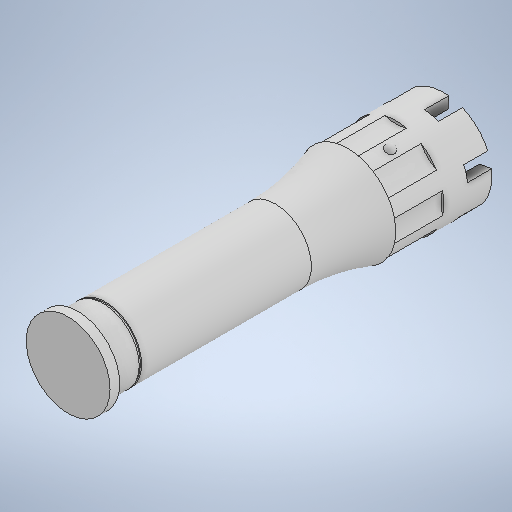
# Autodesk Inventor part: Capsule idea
Saved by Autodesk Inventor 2026.2 (Build 302298000, 298)
## iProperties
Created: 2026-01-17
Part Number: Capsule idea
Material: Generic
Document SubType Name: Modeling
Designer: daryu
Density: 1 g/cm^3
Appearance: Default
Author: daryu
Autodesk Inventor part; units mm, degrees
ref_plane "YZ Plane" through (0, 0, 0) normal (1, 0, 0) x (0, 1, 0)
ref_plane "XZ Plane" through (0, 0, 0) normal (0, 1, 0) x (-1, 0, 0)
ref_plane "XY Plane" through (0, 0, 0) normal (0, 0, 1) x (1, 0, 0)
sketch "Sketch2" plane through (0, 0, 0) normal (1, 0, 0) x (0, 1, 0)
  line L0 (0, 0) -> (15, 0)
  line L1 (15, 0) -> (15, -50)
  line L2 (15, -50) -> (0, -50)
  line L3 (0, -50) -> (0, 0)
  line L4 (7.5, 0) -> (7.5, -50)
  dimension "d0" = 50
  dimension "d1" = 15
  constraints: 10 end point, 2 midpoint, 2 parallel, 2 perpendicular, 1 horizontal
  measures "d0" distance of L0.end L1.end
  measures "d1" distance of L0.start L0.end
revolve "Revolution1" add sketch "Sketch2" angle 360 about axis through (0, 7.5, 0) along (0, 0, -1) contours L0 L1 L2 L4
sketch "Sketch3" plane through (0, 0, 0) normal (1, 0, 0) x (0, 1, 0)
  line L0 (0, -50) -> (15, -50) projected
  line L1 (0, -50) -> (0, -43)
  line L2 (0, 0) -> (0, -50) projected
  arc A0 (-2.5, -58) -> (0, -43) centre (-46.25, -43) ccw
  line L3 (-2.5, -58) -> (0, -58)
  line L4 (0, -58) -> (0, -50)
  line L5 (0, 0) -> (15, 0) projected
  line L6 (7.5, 0) -> (7.5, -50)
  dimension "d5" = 15
  dimension "d6" = 2.5
  dimension "d7" = 8
  constraints: 8 end point, 2 midpoint, 2 point on circle, 1 centre point, 1 horizontal, 1 horizontal alignment, 1 perpendicular, 1 point on line
  measures "d5" vertical distance of L1.end L3.start
  measures "d6" distance of L3.start L3.end
  measures "d7" distance of L0.start L3.end
revolve "Revolution2" add sketch "Sketch3" angle 360 about axis through (0, 7.5, 0) along (0, 0, -1) contours L4 L3 A0 L1
sketch "Sketch4" plane through (0, 7.5, -58) normal (0, 0, -1) x (-1, 0, 0)
  circle A0 centre (0, 0) radius 10 projected
  point P0 (0, -7.5)
extrude "Extrusion1" add sketch "Sketch4" along normal blind 10
sketch "Sketch5" plane through (0, 7.5, -68) normal (0, 0, -1) x (-1, 0, 0)
  circle A0 centre (0, 0) radius 10 projected
  line L0 (0, 0) -> (0, -3.294)
  line L1 (0, 0) -> (7.0711, 7.0711)
  line L2 (0, 0) -> (0, 10)
  arc A1 (5.2892, 8.4867) -> (8.4867, 5.2892) centre (11.8815, 11.8815) ccw
  arc A2 (-2.261, 9.741) -> (2.261, 9.741) centre (0, 16.803) ccw
  arc A3 (-8.4867, 5.2892) -> (-5.2892, 8.4867) centre (-11.8815, 11.8815) ccw
  arc A4 (-9.741, -2.261) -> (-9.741, 2.261) centre (-16.803, 0) ccw
  arc A5 (-5.2892, -8.4867) -> (-8.4867, -5.2892) centre (-11.8815, -11.8815) ccw
  arc A6 (2.261, -9.741) -> (-2.261, -9.741) centre (0, -16.803) ccw
  arc A7 (8.4867, -5.2892) -> (5.2892, -8.4867) centre (11.8815, -11.8815) ccw
  arc A8 (9.741, 2.261) -> (9.741, -2.261) centre (16.803, 0) ccw
  point P0 (0, -7.5)
  point P1 (6.6383, 6.6383)
  point P2 (0, 9.3879)
  point P3 (-6.6383, 6.6383)
  point P4 (-9.3879, 0)
  point P5 (-6.6383, -6.6383)
  point P6 (0, -9.3879)
  point P7 (6.6383, -6.6383)
  point P8 (9.3879, 0)
  point P9 (5.2892, -8.4867)
  point P10 (-2.261, -9.741)
  point P11 (-8.4867, -5.2892)
  point P12 (-9.741, 2.261)
  point P13 (9.741, 2.261)
  point P14 (9.741, -2.261)
  point P15 (2.261, 9.741)
  point P16 (-2.261, 9.741)
  point P17 (-8.4867, 5.2892)
  point P18 (-5.2892, 8.4867)
  dimension "d19" = 3.294
  dimension "d30" = 45
  dimension "d31" = 11.8815
  dimension "d32" = 7.4151
  dimension "d35" = 360
  constraints: 20 point on circle, 8 centre point, 6 end point, 2 vertical, 1 equal length, 1 point on line, 41 other
  measures "d19" distance of L0.start L0.end
  measures "d30" angle of L2 L1
  measures "d31" horizontal distance of L0.start A1.centre
  measures "d32" radius of A1
ref_plane "Work Plane1" through (0, 7.5, 0) normal (0, 0, 1) x (1, 0, 0)
sketch "Sketch6" plane through (0, 7.5, 0) normal (0, 0, 1) x (1, 0, 0)
  circle A0 centre (0, 0) radius 7.5 projected
  circle A1 centre (0, 0) radius 8.7
  point P0 (0, -7.5)
  dimension "d23" = 1.2
  constraints: 1 centre point, 1 vertical alignment
extrude "Extrusion3" add sketch "Sketch6" against normal blind 2
extrude "Extrusion4" cut sketch "Sketch5" against normal blind 10 contours A0 A8 | A1 L1 A0 | A0 A7 | L1 A1 A0 | A0 A6 | A2 L2 A0 | A2 A0 L2 | A0 A5 | A3 A0 | A0 A4
sketch "Sketch7" plane through (0, 7.5, -68) normal (0, 0, -1) x (-1, 0, 0)
  arc A0 (9.741, -2.261) -> (9.741, 2.261) centre (0, 0) ccw projected
  arc A1 (8.4867, -5.2892) -> (9.741, -2.261) centre (0, 0) ccw projected
  arc A2 (5.2892, -8.4867) -> (8.4867, -5.2892) centre (0, 0) ccw projected
  arc A3 (2.261, -9.741) -> (5.2892, -8.4867) centre (0, 0) ccw projected
  arc A4 (-2.261, -9.741) -> (2.261, -9.741) centre (0, 0) ccw projected
  arc A5 (-5.2892, -8.4867) -> (-2.261, -9.741) centre (0, 0) ccw projected
  arc A6 (-8.4867, -5.2892) -> (-5.2892, -8.4867) centre (0, 0) ccw projected
  arc A7 (-9.741, -2.261) -> (-8.4867, -5.2892) centre (0, 0) ccw projected
  arc A8 (-9.741, 2.261) -> (-9.741, -2.261) centre (0, 0) ccw projected
  arc A9 (-8.4867, 5.2892) -> (-9.741, 2.261) centre (0, 0) ccw projected
  arc A10 (-5.2892, 8.4867) -> (-8.4867, 5.2892) centre (0, 0) ccw projected
  arc A11 (-2.261, 9.741) -> (-5.2892, 8.4867) centre (0, 0) ccw projected
  arc A12 (2.261, 9.741) -> (-2.261, 9.741) centre (0, 0) ccw projected
  arc A13 (5.2892, 8.4867) -> (2.261, 9.741) centre (0, 0) ccw projected
  arc A14 (8.4867, 5.2892) -> (5.2892, 8.4867) centre (0, 0) ccw projected
  arc A15 (9.741, 2.261) -> (8.4867, 5.2892) centre (0, 0) ccw projected
  circle A16 centre (0, 0) radius 7.5 projected
  point P0 (0, -7.5)
extrude "Extrusion5" add sketch "Sketch7" along normal blind 10
sketch "Sketch8" plane through (0, 7.5, -78) normal (0, 0, -1) x (-1, 0, 0)
  circle A0 centre (0, 0) radius 7.5 projected
  circle A1 centre (0, 0) radius 10 projected
  line L0 (-4.5, -6) -> (-6.0595, -7.955)
  line L1 (-6, -4.5) -> (-8.1073, -5.8542)
  point P0 (0, -7.5)
  dimension "d41" = 2.5008
  dimension "d42" = 2.5049
  dimension "d43" = 6
  dimension "d44" = 6
  constraints: 4 end point, 4 point on circle
  measures "d41" distance of L0.start L0.end
  measures "d42" distance of L1.start L1.end
  measures "d43" vertical distance of A0.centre L0.start
  measures "d44" horizontal distance of A0.centre L1.start
extrude "Extrusion6" cut sketch "Sketch8" against normal blind 5 contours A0 L0 A1 L1 picked at (-5.972, -6.942)
pattern_circular "Circular Pattern1" count 6 over 360 about axis through (0, 7.5, -58) along (0, 0, -1) of "Extrusion6"
ref_plane "Work Plane2" through (0, 7.5, -7.25) normal (0, 0, 1) x (1, 0, 0)
sketch "Sketch9" plane through (0, 7.5, -7.25) normal (0, 0, 1) x (1, 0, 0)
  circle A0 centre (0, 0) radius 7.5 projected
  circle A1 centre (0, 0) radius 7.25
  point P0 (0, -7.5)
  dimension "d51" = 14.5
  constraints: 1 centre point, 1 vertical alignment
  measures "d51" diameter of A1
extrude "Extrusion7" cut sketch "Sketch9" against normal blind 0.5
ref_plane "Work Plane3" through (3.8268, 16.7388, -58) normal (0.3826834, 0.9238795, 0) x (-0.9238795, 0.3826834, 0)
sketch "Sketch10" plane through (3.8268, 16.7388, -58) normal (0.3826834, 0.9238795, 0) x (-0.9238795, 0.3826834, 0)
  line L0 (-1.6388, 0) -> (1.6388, 0) projected
  line L1 (0, 0) -> (0, -5)
  circle A0 centre (0, -5) radius 1
  line L2 (0, -5) -> (0, -6)
  point P0 (-2.8701, 58)
  point P1 (0, -5)
  point P2 (0, -4)
  dimension "d55" = 2
  dimension "d54" = 5
  constraints: 4 end point, 1 coincident, 1 midpoint, 1 point on line, 1 vertical, 3 other
  measures "d54" distance of L1.start L1.end
revolve "Revolution3" add sketch "Sketch10" angle 360 about axis through (3.8268, 16.7388, -58) along (0, 0, -1) picked at (-0.0798, -5.657) contours L1 L2 A0
scale "Scale1" factors (0.1, 0.1, 0.1) then translate (0, 6.75, -22.8375) bodies 1
body "Solid1"
